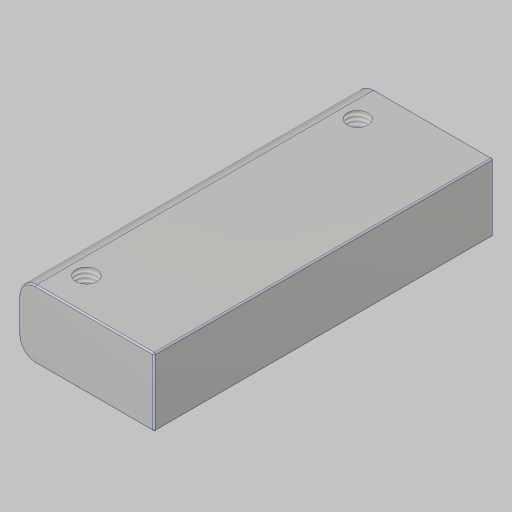
# Autodesk Inventor part: EL2-017
Saved by Autodesk Inventor 2023.5 (Build 275446000, 446)
## iProperties
Created: 2025-01-21
Part Number: EL2-017
Material: Aluminum 6061
Document SubType Name: Modeling
Designer: slick
Density: 2.7 g/cm^3
Appearance: Aluminum - Flat
Author: slick
Autodesk Inventor part; units mm, degrees
ref_plane "YZ Plane" through (0, 0, 0) normal (1, 0, 0) x (0, 1, 0)
ref_plane "XZ Plane" through (0, 0, 0) normal (0, 1, 0) x (-1, 0, 0)
ref_plane "XY Plane" through (0, 0, 0) normal (0, 0, 1) x (1, 0, 0)
sketch "Sketch1" plane through (0, 0, 0) normal (0, 0, 1) x (1, 0, 0)
  line L0 (-12.7, 6.35) -> (12.7, 6.35)
  line L1 (12.7, 6.35) -> (12.7, -6.35)
  line L2 (12.7, -6.35) -> (-12.7, -6.35)
  line L3 (-12.7, -6.35) -> (-12.7, 6.35)
  line L4 (-12.7, 6.35) -> (12.7, -6.35) construction
  line L5 (12.7, 6.35) -> (-12.7, -6.35) construction
  point P0 (0, 0)
  dimension "d0" = 25.4
  dimension "d1" = 12.7
  constraints: 12 end point, 2 midpoint, 2 parallel, 1 horizontal, 1 perpendicular
  measures "d0" distance of L1.end L2.end
  measures "d1" distance of L0.end L1.end
extrude "Extrusion1" add sketch "Sketch1" along normal mid plane 63.5
sketch "Sketch2" plane through (-12.7, 6.35, 31.75) normal (0, 1, 0) x (1, 0, 0)
  line L0 (6.35, 57.15) -> (6.35, 6.35) construction
  line L1 (0, 63.5) -> (0, 0) projected
  point P0 (12.7, 31.75)
  point P1 (6.35, 31.75)
  dimension "d4" = 50.8
  dimension "d5" = 6.35
  constraints: 2 end point, 1 horizontal alignment, 1 midpoint, 1 vertical, 1 vertical alignment
  measures "d4" distance of L0.start L0.end
  measures "d5" distance between parallel lines of L1 L0
hole "Hole1" at (-6.35, 6.35, 25.4) at (-6.35, 6.35, -25.4) direction (0, -1, 0) diameter 3.9624 end through all thread size "10-32 UNF" class "2B" standard "ANSI Unified Screw Threads"
fillet "Fillet1" radius 3.175 2 edges at (-12.7, 6.35, 0) (-12.7, -6.35, 0)
fillet "Fillet2" radius 0.254 14 edges at (-11.7701, 5.4201, 31.75) (-12.7, 0, 31.75) (-11.7701, -5.4201, 31.75) (1.5875, -6.35, 31.75) (1.5875, 6.35, 31.75) (12.7, 6.35, 0) (12.7, -6.35, 0) (12.7, 0, -31.75) (12.7, 0, 31.75) (-11.7701, 5.4201, -31.75) (-12.7, 0, -31.75) (-11.7701, -5.4201, -31.75) (1.5875, -6.35, -31.75) (1.5875, 6.35, -31.75)
body "Solid1"
